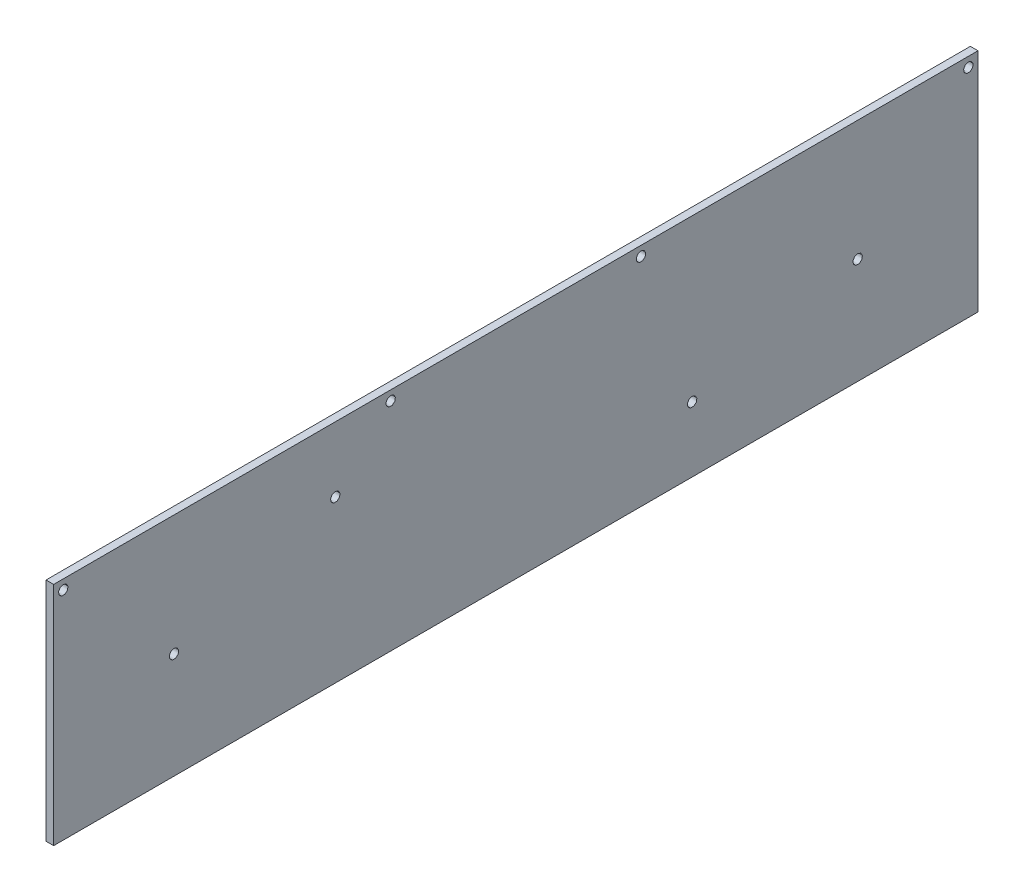
# Autodesk Inventor part: OutsideChassiPlate4.0
Saved by Autodesk Inventor 2023 (Build 270158000, 158)
## iProperties
Created: 2022-10-05
Part Number: OutsideChassiPlate4.0
Material: Generic
Document SubType Name: Modeling
Designer: deli
Density: 1 g/cm^3
Appearance: Default
Author: deli
Autodesk Inventor part; units mm, degrees
ref_plane "YZ Plane" through (0, 0, 0) normal (1, 0, 0) x (0, 1, 0)
ref_plane "XZ Plane" through (0, 0, 0) normal (0, 1, 0) x (-1, 0, 0)
ref_plane "XY Plane" through (0, 0, 0) normal (0, 0, 1) x (1, 0, 0)
sketch "Sketch1" plane through (0, 0, 0) normal (1, 0, 0) x (0, 1, 0)
  line L0 (-90, 4) -> (-90, -380) projected
  line L1 (-90, -380) -> (4, -380) projected
  line L2 (4, -380) -> (4, 4) projected
  line L3 (4, 4) -> (-90, 4) projected
  circle A0 centre (0, -240) radius 2 projected
  circle A1 centre (0, -376) radius 2 projected
  circle A2 centre (-46.95, -203.128) radius 1.9844 projected
  circle A3 centre (-78.95, -187.128) radius 1.9844 projected
  circle A4 centre (-23.05, -113.0058) radius 2 projected
  circle A5 centre (-39.05, -171.1088) radius 1.9844 projected
  circle A6 centre (-39.05, -187.1088) radius 1.9844 projected
  circle A7 centre (-7.05, -187.1088) radius 1.9844 projected
  circle A8 centre (-7.05, -171.1088) radius 1.9844 projected
  circle A9 centre (0, 0) radius 2 projected
  circle A10 centre (-46, -330) radius 2 projected
  circle A11 centre (-46, -46) radius 2 projected
  circle A12 centre (-78.95, -203.128) radius 1.9844 projected
  circle A13 centre (-46.95, -187.128) radius 1.9844 projected
  circle A14 centre (-62.95, -261.231) radius 2 projected
  circle A15 centre (0, -136) radius 2 projected
extrude "Extrusion1" add sketch "Sketch1" along normal blind 3.175 contours L3 L2 L1 L0 | A2 | A3 | A5 | A6 | A7 | A8 | A12 | A13
body "Solid1"
